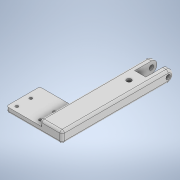
# Autodesk Inventor part: lever
Saved by Autodesk Inventor 2020 (Build 240168000, 168)
## iProperties
Created: 2019-11-14
Part Number: lever
Material: Generic
Document SubType Name: Modeling
Designer: bzs3334
Density: 1 g/cm^3
Appearance: Default
Author: bzs3334
Autodesk Inventor part; units mm, degrees
ref_plane "YZ Plane" through (0, 0, 0) normal (1, 0, 0) x (0, 1, 0)
ref_plane "XZ Plane" through (0, 0, 0) normal (0, 1, 0) x (-1, 0, 0)
ref_plane "XY Plane" through (0, 0, 0) normal (0, 0, 1) x (1, 0, 0)
sketch "Sketch1" plane through (0, 0, 0) normal (0, 1, 0) x (-1, 0, 0)
  line L0 (10, 0) -> (-10, 0)
  line L1 (-10, 0) -> (-10, 100)
  line L2 (-10, 100) -> (10, 100)
  line L3 (10, 100) -> (10, 0)
  line L4 (5, 0) -> (-5, 0)
  line L5 (-5, 0) -> (-5, 20)
  line L6 (-5, 20) -> (5, 20)
  line L7 (5, 20) -> (5, 0)
  line L8 (50, 0) -> (-20, 0) projected
  line L9 (10, 100) -> (40, 100)
  line L10 (40, 100) -> (40, 70)
  line L11 (40, 70) -> (10, 70)
  line L12 (10, 70) -> (10, 100)
  circle A0 centre (35, 95.5) radius 1.25
  circle A1 centre (14, 95.5) radius 1.25
  circle A2 centre (35, 83) radius 1.25
  circle A3 centre (14, 83) radius 1.25
  point P0 (0, 0)
  point P1 (-5, 0)
  dimension "d0" = 20
  dimension "d1" = 10
  dimension "d2" = 100
  dimension "d3" = 20
  dimension "d4" = 5
  dimension "d5" = 5
  dimension "d8" = 30
  dimension "d9" = 30
  dimension "d10" = 2.5
  dimension "d11" = 4.5
  dimension "d12" = 5
  dimension "d15" = 21
  dimension "d18" = 12.5
  constraints: 24 end point, 6 parallel, 4 centre point, 4 horizontal, 3 perpendicular, 1 collinear, 1 point on line, 1 vertical, 6 other
  measures "d0" distance between parallel lines of L1 L3
  measures "d1" distance from line of point (0, 0) L3
  measures "d2" distance of L0.end L1.end
  measures "d3" distance between parallel lines of L0 L6
  measures "d4" distance between parallel lines of L3 L7
  measures "d5" distance between parallel lines of L5 L1
  measures "d8" distance of L9.end L10.end
  measures "d9" distance of L10.end L11.end
  measures "d10" diameter of A0
  measures "d11" distance from line of L9 A0.centre
  measures "d12" distance from line of L10 A0.centre
  measures "d15" distance of A0.centre A1.centre
  measures "d18" distance of A0.centre A2.centre
extrude "Extrusion1" add sketch "Sketch1" along normal blind 10 contours L0 L7 L6 L5 L1 L2 L3
extrude "Extrusion2" add sketch "Sketch1" along normal blind 5 contours L3 L9 L10 L11
fillet "Fillet1" radius 5 4 edges at (7.5, 10, 0) (7.5, 0, 0) (-7.5, 0, 0) (-7.5, 10, 0)
sketch "Sketch2" plane through (10, 0, 100) normal (1, 0, 0) x (0, 0, -1)
  circle A0 centre (95, 5) radius 2
  arc A1 (95, 0) -> (95, 10) centre (95, 5) ccw projected
  line L0 (0, 10) -> (95, 10) projected
  line L1 (0, 0) -> (0, 10) projected
  line L2 (0, 0) -> (95, 0) projected
  point P0 (100, 0)
  dimension "d24" = 4
  constraints: 1 centre point, 1 concentric
  measures "d24" diameter of A0
extrude "Extrusion3" cut sketch "Sketch2" against normal blind 81 contours A0
fillet "Fillet3" radius 2 2 edges at (-40, 2.5, 100) (-40, 2.5, 70)
fillet "Fillet4" radius 2 10 edges at (-10, 1.4644, 1.4644) (-10, 5, 0) (-10, 8.5356, 1.4644) (-10, 0, 37.4999) (-10, 10, 52.4999) (10, 5, 0) (10, 1.4644, 1.4644) (10, 8.5356, 1.4644) (10, 0, 52.4999) (10, 10, 52.4999)
fillet "Fillet5" radius 2 12 edges at (9.4142, 9.4142, 100) (10, 5, 100) (9.4142, 0.5858, 100) (-15, 0, 100) (-39.4142, 0, 99.4142) (-40, 0, 85) (-39.4142, 0, 70.5858) (-9, 0, 70) (-24, 0, 70) (-9.4142, 9.4142, 100) (-10, 6.5, 100) (0, 10, 100)
sketch "Sketch3" plane through (0, 10, 0) normal (0, 1, 0) x (1, 0, 0)
  line L0 (8, -98) -> (-8, -98) projected
  line L1 (8, -5) -> (8, -98) projected
  line L2 (5, -5) -> (8, -5) projected
  line L3 (5, -5) -> (5, -20) projected
  line L4 (5, -20) -> (-5, -20) projected
  line L5 (-5, -20) -> (-5, -5) projected
  line L6 (-8, -5) -> (-5, -5) projected
  line L7 (-8, -98) -> (-8, -5) projected
  line L8 (0, 20) -> (0, -120) projected
  circle A0 centre (0, -30) radius 2.1
  point P0 (0, 0)
  dimension "d31" = 4.2
  dimension "d32" = 10
  constraints: 1 centre point, 1 point on line
  measures "d31" diameter of A0
  measures "d32" distance from line of L4 A0.centre
extrude "Extrusion4" cut sketch "Sketch3" against normal blind 81 contours A0 L8 | L8 A0
equation "\"d1\" = 0.5 * d0"
equation "\"d5\" = d4"
body "Solid1"
